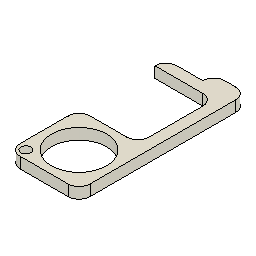
covid v2 (Autodesk Fusion 360 design; units mm, degrees)
Autodesk Fusion 360 part; units mm, degrees
sketch "Sketch1" plane through (0, 0, 0) normal (0, 1, 0) x (1, 0, 0)
  line L0 (5, 0) -> (26.75, 0)
  line L1 (31.75, 5) -> (31.75, 76.2)
  line L2 (26.75, 76.2) -> (21.75, 76.2)
  line L3 (16.75, 71.2) -> (16.75, 71.2)
  line L4 (16.75, 71.2) -> (5, 71.2)
  line L5 (0, 66.2) -> (0, 66.2)
  line L6 (31.75, 71.2) -> (31.75, 66.2)
  line L7 (0, 66.2) -> (21.75, 66.2)
  line L8 (26.75, 61.2) -> (26.75, 36.75)
  line L9 (21.75, 31.75) -> (5, 31.75)
  line L10 (0, 26.75) -> (0, 5)
  arc A0 (21.75, 76.2) -> (16.75, 71.2) centre (21.75, 71.2) ccw
  arc A1 (31.75, 71.2) -> (26.75, 76.2) centre (26.75, 71.2) ccw
  arc A2 (5, 71.2) -> (0, 66.2) centre (5, 66.2) ccw
  arc A3 (26.75, 61.2) -> (21.75, 66.2) centre (21.75, 61.2) ccw
  arc A4 (21.75, 31.75) -> (26.75, 36.75) centre (21.75, 36.75) ccw
  arc A5 (5, 31.75) -> (0, 26.75) centre (5, 26.75) ccw
  arc A6 (0, 5) -> (5, 0) centre (5, 5) ccw
  arc A7 (26.75, 0) -> (31.75, 5) centre (26.75, 5) ccw
  circle A8 centre (15.875, 15.875) radius 12.5
  circle A9 centre (3.801, 3.801) radius 2.25
  dimension "d12" = 25
  constraint horizontal L0
  constraint perpendicular L0 L1
  constraint perpendicular L1 L2
  constraint perpendicular L2 L6
  constraint perpendicular L8 L9
  constraint perpendicular L0 L10
  constraint tangent L2 A0
  constraint coincident L1.end L6
  constraint coincident L1.end L2
  constraint tangent L6 A1
  constraint tangent L2 A1
  constraint tangent L4 A2
  constraint equal A1 A2
  constraint tangent L7 A3
  constraint tangent L8 A3
  constraint equal A1 A3
  constraint tangent L8 A4
  constraint tangent L9 A4
  constraint equal A1 A4
  constraint tangent L9 A5
  constraint equal A1 A5
  constraint tangent L0 A6
  constraint equal A1 A6
  constraint tangent L0 A7
  constraint tangent L1 A7
  constraint equal A1 A7
  measures "d12" diameter of A8
extrude "Extrude1" add sketch "Sketch1" along normal blind 5
sketch "Sketch2" plane through (0, 0, 0) normal (1, 0, 0) x (0, 0, -1)
